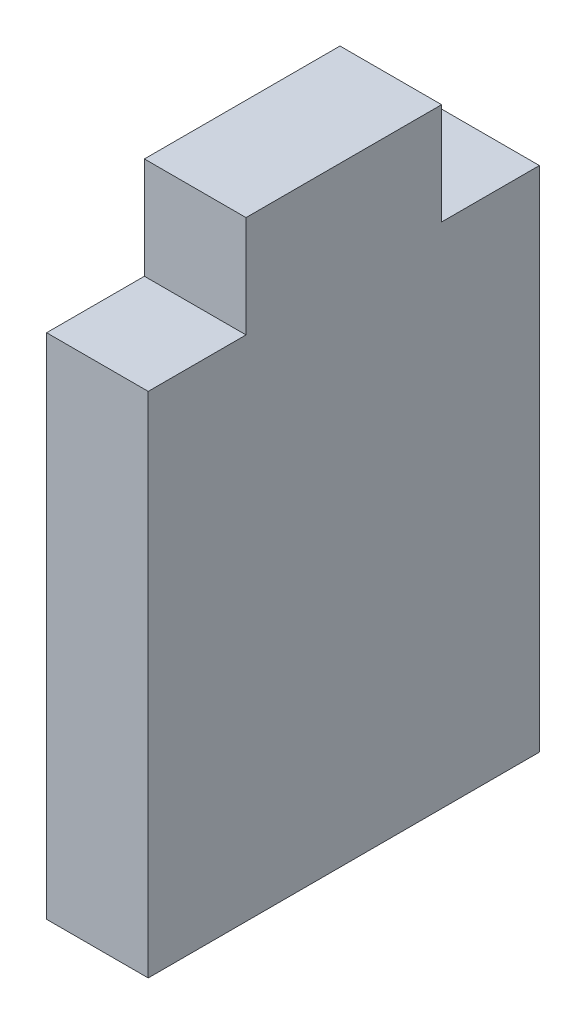
# Autodesk Inventor part: HalterungServosHochSeitlich
Saved by Autodesk Inventor 2020.3 (Build 243373010, 373A)
## iProperties
Created: 2020-12-10
Part Number: HalterungServosHochSeitlich
Material: Generisch
Document SubType Name: Modeling
Designer: Stefan
Density: 1 g/cm^3
Appearance: Vorgabe
Author: Stefan
Autodesk Inventor part; units mm, degrees
ref_plane "YZ Plane" through (0, 0, 0) normal (1, 0, 0) x (0, 1, 0)
ref_plane "XZ Plane" through (0, 0, 0) normal (0, 1, 0) x (-1, 0, 0)
ref_plane "XY Plane" through (0, 0, 0) normal (0, 0, 1) x (1, 0, 0)
sketch "Skizze1" plane through (0, 0, 0) normal (1, 0, 0) x (0, 1, 0)
  line L0 (0, 0) -> (-50, 0)
  line L1 (-50, 0) -> (-50, 38.5)
  line L2 (-50, 38.5) -> (0, 38.5)
  line L3 (0, 28.875) -> (10, 28.875)
  line L4 (10, 28.875) -> (10, 9.625)
  line L5 (10, 9.625) -> (0, 9.625)
  line L6 (0, 38.5) -> (0, 28.875)
  line L7 (0, 9.625) -> (0, 0)
  dimension "d0" = 50
  dimension "d1" = 38.5
  dimension "d2" = 10
  dimension "d3" = 19.25
  dimension "d4" = 9.625
  constraints: 16 end point, 4 parallel, 2 horizontal, 2 perpendicular
  measures "d0" distance of L1.end L2.end
  measures "d1" distance of L2.end L0.start
  measures "d2" distance of L4.end L5.end
  measures "d3" distance of L3.end L4.end
  measures "d4" distance between parallel lines of L2 L3
extrude "Extrusion1" add sketch "Skizze1" along normal blind 10
